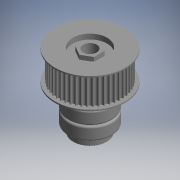
# Autodesk Inventor part: SLZ_63_Riemengetribe#
Saved by Autodesk Inventor 2017.3 (Build 213256000, 256)
## iProperties
Part Number: SLZ_63_Riemengetribe#
Material: Generic
Catalog Web Link: www.cadenas.de
Description: Riemengetr SLZ63-Control-Tec
Vendor: ROSEKRIEGER
Document SubType Name: Modeling
Designer: partserver
Manufacturer: ROSEKRIEGER
Mass: 220.102 g
Surface Area: 442.703 cm^2
Volume: 220.102 cm^3
Density: 1 g/cm^3
Appearance: PSOLRGB-175-175-175
Category: PARTsolutions
Company: ROSEKRIEGER
Title: SLZ_63_Riemengetribe#
Author: Cadenas PARTsolutions
Comments: Control-Tec
PSOL_IDENT_0: {$CADENAS_DATA\23d-libs\rose_krieger\linearkomponenten\pool_lineartechnik\_hubsaeule_zyliinder\elekt
PSOL_IDENT_1: rozylinder\elekzyl_slz63\parts\slz63_plfl_riemengetribe.prj},192 {VTYP=3D},{NB=SLZ_63_Riemengetribe#
PSOL_IDENT_2: },{LINA=SLZ_63_Riemengetribe#},{NN=Riemengetr SLZ63},{DATE=02.12.2020 11:16:20},{GEOMDATE=22.06.2016
PSOL_IDENT_3: 13:04:22},{VERSION=},{LINEID=10},{WBVAR=},{WBNUMERIC=}  {NB=SLZ_63_Riemengetribe#},{LINA=SLZ_63_Rie
PSOL_IDENT_4: mengetribe#},{KT=DUMMY},{IDNR=},{CODE=TQ3},{ARTIKEL=Elektrozylinder },{TYPE=SLZ 63 KG P PL},{BEST=SL
PSOL_IDENT_5: Z_63_Riemengetribe},{VARIANTE=PL},{SPINDEL=KG 25x10},{SPINDELCODE=3.000},{SCHUTZARTVIS=IP54},{SCHUTZ
PSOL_IDENT_6: ART=1},{HUB1=0,[0:100]},{HINWEINBAUX=Hub + 288,5 mm},{DUMMYDURCH=10.000},{DUMMYLAENG=20.000},{HILFEH
PSOL_IDENT_7: UB=105},{LAENDOPPROFIL=184.500},{RF=1.000},{GRUNDKOE=288.500},{A=100},{B=80},{C=100},{D=125},{E=238}
PSOL_IDENT_8: ,{F=40},{G=M16x1.5},{H=104},{K=125},{L=105},{M=48},{N=56.5},{O=86},{P=18.5},{PPATH=sbl_lz70p_plfl.pr
PSOL_IDENT_9: j}
NB: SLZ_63_Riemengetribe#
NN: Riemengetr SLZ63
NT: Control-Tec
NBSYN: $BEST.#
LINA: SLZ_63_Riemengetribe#
CATALOG: RK Rose+Krieger
BEST: SLZ_63_Riemengetribe
VARIANTE: PL
SPINDEL: KG 25x10
SPINDELCODE: 3
SCHUTZARTVIS: IP54
SCHUTZART: 1
HUB1: 0,[0:100]
HINWEINBAUX: Hub + 288,5 mm
HILFEHUB: 105
LAENDOPPROFIL: 184.5
RF: 1
GRUNDKOE: 288.5
A: 100
B: 80
C: 100
D: 125
E: 238
F: 40
G: M16x1.5
H: 104
K: 125
L: 105
M: 48
N: 56.5
O: 86
P: 18.5
SUPPLIER: ROSEKRIEGER
ARTICLENO: SLZ_63_Riemengetribe#
BOMINFO: SLZ_63_Riemengetribe#
CREATOR: CADENAS GmbH
Autodesk Inventor part; units mm, degrees
sketch "Sketch_3" plane through (0, 0, 0) normal (1, 0, 0) x (0, 0, -1)
  line L0 (0, 0) -> (-87, 0)
  line L1 (-87, 19.5) -> (-87, 10)
  line L2 (-87, 10) -> (-36, 10)
  line L3 (-36, 10) -> (-36, 8)
  line L4 (-36, 8) -> (-1, 8)
  line L5 (-1, 8) -> (-1, 12.975)
  line L6 (-1, 12.975) -> (-6, 12.975)
  line L7 (-6, 12.975) -> (-6, 20.25)
  line L8 (-6, 20.25) -> (0, 20.25)
  line L9 (0, 20.25) -> (0, 41.5)
  line L10 (0, 41.5) -> (-1.5, 41.5)
  line L11 (-1.5, 41.5) -> (-1.5, 24)
  line L12 (-1.5, 24) -> (-34.5, 24)
  line L13 (-34.5, 24) -> (-34.5, 41.5)
  line L14 (-34.5, 41.5) -> (-36, 41.5)
  line L15 (-36, 41.5) -> (-36, 20)
  line L16 (-36, 20) -> (-38, 20)
  line L17 (-38, 20) -> (-38, 26)
  line L18 (-38, 26) -> (-39, 27)
  line L19 (-39, 27) -> (-44.5, 27)
  line L20 (-44.5, 27) -> (-45.5, 26)
  line L21 (-45.5, 26) -> (-45.5, 25.5)
  line L22 (-45.5, 25.5) -> (-46.5, 25.5)
  line L23 (-46.5, 25.5) -> (-47, 25)
  line L24 (-47, 25) -> (-47, 24)
  arc A0 (-47, 24) -> (-49, 26) centre (-49, 24) ccw
  line L25 (-49, 26) -> (-60, 26)
  arc A1 (-60, 26) -> (-62, 24) centre (-60, 24) ccw
  line L26 (-62, 24) -> (-62, 20)
  line L27 (-62, 20) -> (-63, 20)
  line L28 (-63, 20) -> (-63, 24)
  arc A2 (-63, 24) -> (-65, 26) centre (-65, 24) ccw
  line L29 (-65, 26) -> (-76, 26)
  arc A3 (-76, 26) -> (-78, 24) centre (-76, 24) ccw
  line L30 (-78, 24) -> (-78, 15)
  line L31 (-78, 15) -> (-79, 15)
  line L32 (-79, 15) -> (-79, 19.5)
  line L33 (-79, 19.5) -> (-79.5, 20)
  line L34 (-79.5, 20) -> (-86.5, 20)
  line L35 (-86.5, 20) -> (-87, 19.5)
  constraints: 72 end point, 8 point on circle, 4 centre point
revolve "Revolution1" add sketch "Sketch_3" angle 360 about axis through (0, 0, 0) along (0, 0, -1)
sketch "Sketch_1" plane through (0, 0, 1.5) normal (0, 0, 1) x (1, 0, 0)
  arc A0 (-37.2613, -1.9994) -> (-37.5535, -2.3178) centre (-37.2541, -2.2993) ccw
  arc A1 (-37.5535, -2.3178) -> (-37.5348, -2.6037) centre (0, 0) ccw
  arc A2 (-37.5348, -2.6037) -> (-37.2035, -2.8812) centre (-37.2355, -2.583) ccw
  arc A3 (-36.6815, -6.8459) -> (-37.2035, -2.8812) centre (-36.9898, -4.8698) ccw
  arc A4 (-36.6815, -6.8459) -> (-36.9297, -7.1997) centre (-36.6353, -7.1423) ccw
  arc A5 (-36.9297, -7.1997) -> (-36.8738, -7.4807) centre (0, 0) ccw
  arc A6 (-36.8738, -7.4807) -> (-36.5091, -7.7126) centre (-36.5798, -7.4211) ccw
  arc A7 (-35.4741, -11.5752) -> (-36.5091, -7.7126) centre (-36.0377, -9.6563) ccw
  arc A8 (-35.4741, -11.5752) -> (-35.674, -11.9584) centre (-35.3896, -11.8631) ccw
  arc A9 (-35.674, -11.9584) -> (-35.5819, -12.2297) centre (0, 0) ccw
  arc A10 (-35.5819, -12.2297) -> (-35.1901, -12.412) centre (-35.2982, -12.1322) ccw
  arc A11 (-33.6598, -16.1065) -> (-35.1901, -12.412) centre (-34.469, -14.2775) ccw
  arc A12 (-33.6598, -16.1065) -> (-33.808, -16.5125) centre (-33.5384, -16.3808) ccw
  arc A13 (-33.808, -16.5125) -> (-33.6812, -16.7695) centre (0, 0) ccw
  arc A14 (-33.6812, -16.7695) -> (-33.2689, -16.8991) centre (-33.4127, -16.6358) ccw
  arc A15 (-31.2695, -20.3622) -> (-33.2689, -16.8991) centre (-32.3105, -18.6545) ccw
  arc A16 (-31.2695, -20.3622) -> (-31.3634, -20.7841) centre (-31.1133, -20.6183) ccw
  arc A17 (-31.3634, -20.7841) -> (-31.2042, -21.0223) centre (0, 0) ccw
  arc A18 (-31.2042, -21.0223) -> (-30.7785, -21.097) centre (-30.9554, -20.8547) ccw
  arc A19 (-28.3442, -24.2695) -> (-30.7785, -21.097) centre (-29.5992, -22.7123) ccw
  arc A20 (-28.3442, -24.2695) -> (-28.3822, -24.7) centre (-28.1559, -24.5031) ccw
  arc A21 (-28.3822, -24.7) -> (-28.1933, -24.9154) centre (0, 0) ccw
  arc A22 (-28.1933, -24.9154) -> (-27.7615, -24.9339) centre (-27.9685, -24.7168) ccw
  arc A23 (-24.9339, -27.7615) -> (-27.7615, -24.9339) centre (-26.3814, -26.3814) ccw
  arc A24 (-24.9339, -27.7615) -> (-24.9154, -28.1933) centre (-24.7168, -27.9685) ccw
  arc A25 (-24.9154, -28.1933) -> (-24.7, -28.3822) centre (0, 0) ccw
  arc A26 (-24.7, -28.3822) -> (-24.2695, -28.3442) centre (-24.5031, -28.1559) ccw
  arc A27 (-21.097, -30.7785) -> (-24.2695, -28.3442) centre (-22.7123, -29.5992) ccw
  arc A28 (-21.097, -30.7785) -> (-21.0223, -31.2042) centre (-20.8547, -30.9554) ccw
  arc A29 (-21.0223, -31.2042) -> (-20.7841, -31.3634) centre (0, 0) ccw
  arc A30 (-20.7841, -31.3634) -> (-20.3622, -31.2695) centre (-20.6183, -31.1133) ccw
  arc A31 (-16.8991, -33.2689) -> (-20.3622, -31.2695) centre (-18.6545, -32.3105) ccw
  arc A32 (-16.8991, -33.2689) -> (-16.7695, -33.6812) centre (-16.6358, -33.4127) ccw
  arc A33 (-16.7695, -33.6812) -> (-16.5125, -33.808) centre (0, 0) ccw
  arc A34 (-16.5125, -33.808) -> (-16.1065, -33.6598) centre (-16.3808, -33.5384) ccw
  arc A35 (-12.412, -35.1901) -> (-16.1065, -33.6598) centre (-14.2775, -34.469) ccw
  arc A36 (-12.412, -35.1901) -> (-12.2297, -35.5819) centre (-12.1322, -35.2982) ccw
  arc A37 (-12.2297, -35.5819) -> (-11.9584, -35.674) centre (0, 0) ccw
  arc A38 (-11.9584, -35.674) -> (-11.5752, -35.4741) centre (-11.8631, -35.3896) ccw
  arc A39 (-7.7126, -36.5091) -> (-11.5752, -35.4741) centre (-9.6563, -36.0377) ccw
  arc A40 (-7.7126, -36.5091) -> (-7.4807, -36.8738) centre (-7.4211, -36.5798) ccw
  arc A41 (-7.4807, -36.8738) -> (-7.1997, -36.9297) centre (0, 0) ccw
  arc A42 (-7.1997, -36.9297) -> (-6.8459, -36.6815) centre (-7.1423, -36.6353) ccw
  arc A43 (-2.8812, -37.2035) -> (-6.8459, -36.6815) centre (-4.8698, -36.9898) ccw
  arc A44 (-2.8812, -37.2035) -> (-2.6037, -37.5348) centre (-2.583, -37.2355) ccw
  arc A45 (-2.6037, -37.5348) -> (-2.3178, -37.5535) centre (0, 0) ccw
  arc A46 (-2.3178, -37.5535) -> (-1.9994, -37.2613) centre (-2.2993, -37.2541) ccw
  arc A47 (1.9994, -37.2613) -> (-1.9994, -37.2613) centre (0, -37.309) ccw
  arc A48 (1.9994, -37.2613) -> (2.3178, -37.5535) centre (2.2993, -37.2541) ccw
  arc A49 (2.3178, -37.5535) -> (2.6037, -37.5348) centre (0, 0) ccw
  arc A50 (2.6037, -37.5348) -> (2.8812, -37.2035) centre (2.583, -37.2355) ccw
  arc A51 (6.8459, -36.6815) -> (2.8812, -37.2035) centre (4.8698, -36.9898) ccw
  arc A52 (6.8459, -36.6815) -> (7.1997, -36.9297) centre (7.1423, -36.6353) ccw
  arc A53 (7.1997, -36.9297) -> (7.4807, -36.8738) centre (0, 0) ccw
  arc A54 (7.4807, -36.8738) -> (7.7126, -36.5091) centre (7.4211, -36.5798) ccw
  arc A55 (11.5752, -35.4741) -> (7.7126, -36.5091) centre (9.6563, -36.0377) ccw
  arc A56 (11.5752, -35.4741) -> (11.9584, -35.674) centre (11.8631, -35.3896) ccw
  arc A57 (11.9584, -35.674) -> (12.2297, -35.5819) centre (0, 0) ccw
  arc A58 (12.2297, -35.5819) -> (12.412, -35.1901) centre (12.1322, -35.2982) ccw
  arc A59 (16.1065, -33.6598) -> (12.412, -35.1901) centre (14.2775, -34.469) ccw
  arc A60 (16.1065, -33.6598) -> (16.5125, -33.808) centre (16.3808, -33.5384) ccw
  arc A61 (16.5125, -33.808) -> (16.7695, -33.6812) centre (0, 0) ccw
  arc A62 (16.7695, -33.6812) -> (16.8991, -33.2689) centre (16.6358, -33.4127) ccw
  arc A63 (20.3622, -31.2695) -> (16.8991, -33.2689) centre (18.6545, -32.3105) ccw
  arc A64 (20.3622, -31.2695) -> (20.7841, -31.3634) centre (20.6183, -31.1133) ccw
  arc A65 (20.7841, -31.3634) -> (21.0223, -31.2042) centre (0, 0) ccw
  arc A66 (21.0223, -31.2042) -> (21.097, -30.7785) centre (20.8547, -30.9554) ccw
  arc A67 (24.2695, -28.3442) -> (21.097, -30.7785) centre (22.7123, -29.5992) ccw
  arc A68 (24.2695, -28.3442) -> (24.7, -28.3822) centre (24.5031, -28.1559) ccw
  arc A69 (24.7, -28.3822) -> (24.9154, -28.1933) centre (0, 0) ccw
  arc A70 (24.9154, -28.1933) -> (24.9339, -27.7615) centre (24.7168, -27.9685) ccw
  arc A71 (27.7615, -24.9339) -> (24.9339, -27.7615) centre (26.3814, -26.3814) ccw
  arc A72 (27.7615, -24.9339) -> (28.1933, -24.9154) centre (27.9685, -24.7168) ccw
  arc A73 (28.1933, -24.9154) -> (28.3822, -24.7) centre (0, 0) ccw
  arc A74 (28.3822, -24.7) -> (28.3442, -24.2695) centre (28.1559, -24.5031) ccw
  arc A75 (30.7785, -21.097) -> (28.3442, -24.2695) centre (29.5992, -22.7123) ccw
  arc A76 (30.7785, -21.097) -> (31.2042, -21.0223) centre (30.9554, -20.8547) ccw
  arc A77 (31.2042, -21.0223) -> (31.3634, -20.7841) centre (0, 0) ccw
  arc A78 (31.3634, -20.7841) -> (31.2695, -20.3622) centre (31.1133, -20.6183) ccw
  arc A79 (33.2689, -16.8991) -> (31.2695, -20.3622) centre (32.3105, -18.6545) ccw
  arc A80 (33.2689, -16.8991) -> (33.6812, -16.7695) centre (33.4127, -16.6358) ccw
  arc A81 (33.6812, -16.7695) -> (33.808, -16.5125) centre (0, 0) ccw
  arc A82 (33.808, -16.5125) -> (33.6598, -16.1065) centre (33.5384, -16.3808) ccw
  arc A83 (35.1901, -12.412) -> (33.6598, -16.1065) centre (34.469, -14.2775) ccw
  arc A84 (35.1901, -12.412) -> (35.5819, -12.2297) centre (35.2982, -12.1322) ccw
  arc A85 (35.5819, -12.2297) -> (35.674, -11.9584) centre (0, 0) ccw
  arc A86 (35.674, -11.9584) -> (35.4741, -11.5752) centre (35.3896, -11.8631) ccw
  arc A87 (36.5091, -7.7126) -> (35.4741, -11.5752) centre (36.0377, -9.6563) ccw
  arc A88 (36.5091, -7.7126) -> (36.8738, -7.4807) centre (36.5798, -7.4211) ccw
  arc A89 (36.8738, -7.4807) -> (36.9297, -7.1997) centre (0, 0) ccw
  arc A90 (36.9297, -7.1997) -> (36.6815, -6.8459) centre (36.6353, -7.1423) ccw
  arc A91 (37.2035, -2.8812) -> (36.6815, -6.8459) centre (36.9898, -4.8698) ccw
  arc A92 (37.2035, -2.8812) -> (37.5348, -2.6037) centre (37.2355, -2.583) ccw
  arc A93 (37.5348, -2.6037) -> (37.5535, -2.3178) centre (0, 0) ccw
  arc A94 (37.5535, -2.3178) -> (37.2613, -1.9994) centre (37.2541, -2.2993) ccw
  arc A95 (37.2613, 1.9994) -> (37.2613, -1.9994) centre (37.309, 0) ccw
  arc A96 (37.2613, 1.9994) -> (37.5535, 2.3178) centre (37.2541, 2.2993) ccw
  arc A97 (37.5535, 2.3178) -> (37.5348, 2.6037) centre (0, 0) ccw
  arc A98 (37.5348, 2.6037) -> (37.2035, 2.8812) centre (37.2355, 2.583) ccw
  arc A99 (36.6815, 6.8459) -> (37.2035, 2.8812) centre (36.9898, 4.8698) ccw
  arc A100 (36.6815, 6.8459) -> (36.9297, 7.1997) centre (36.6353, 7.1423) ccw
  arc A101 (36.9297, 7.1997) -> (36.8738, 7.4807) centre (0, 0) ccw
  arc A102 (36.8738, 7.4807) -> (36.5091, 7.7126) centre (36.5798, 7.4211) ccw
  arc A103 (35.4741, 11.5752) -> (36.5091, 7.7126) centre (36.0377, 9.6563) ccw
  arc A104 (35.4741, 11.5752) -> (35.674, 11.9584) centre (35.3896, 11.8631) ccw
  arc A105 (35.674, 11.9584) -> (35.5819, 12.2297) centre (0, 0) ccw
  arc A106 (35.5819, 12.2297) -> (35.1901, 12.412) centre (35.2982, 12.1322) ccw
  arc A107 (33.6598, 16.1065) -> (35.1901, 12.412) centre (34.469, 14.2775) ccw
  arc A108 (33.6598, 16.1065) -> (33.808, 16.5125) centre (33.5384, 16.3808) ccw
  arc A109 (33.808, 16.5125) -> (33.6812, 16.7695) centre (0, 0) ccw
  arc A110 (33.6812, 16.7695) -> (33.2689, 16.8991) centre (33.4127, 16.6358) ccw
  arc A111 (31.2695, 20.3622) -> (33.2689, 16.8991) centre (32.3105, 18.6545) ccw
  arc A112 (31.2695, 20.3622) -> (31.3634, 20.7841) centre (31.1133, 20.6183) ccw
  arc A113 (31.3634, 20.7841) -> (31.2042, 21.0223) centre (0, 0) ccw
  arc A114 (31.2042, 21.0223) -> (30.7785, 21.097) centre (30.9554, 20.8547) ccw
  arc A115 (28.3442, 24.2695) -> (30.7785, 21.097) centre (29.5992, 22.7123) ccw
  arc A116 (28.3442, 24.2695) -> (28.3822, 24.7) centre (28.1559, 24.5031) ccw
  arc A117 (28.3822, 24.7) -> (28.1933, 24.9154) centre (0, 0) ccw
  arc A118 (28.1933, 24.9154) -> (27.7615, 24.9339) centre (27.9685, 24.7168) ccw
  arc A119 (24.9339, 27.7615) -> (27.7615, 24.9339) centre (26.3814, 26.3814) ccw
  arc A120 (24.9339, 27.7615) -> (24.9154, 28.1933) centre (24.7168, 27.9685) ccw
  arc A121 (24.9154, 28.1933) -> (24.7, 28.3822) centre (0, 0) ccw
  arc A122 (24.7, 28.3822) -> (24.2695, 28.3442) centre (24.5031, 28.1559) ccw
  arc A123 (21.097, 30.7785) -> (24.2695, 28.3442) centre (22.7123, 29.5992) ccw
  arc A124 (21.097, 30.7785) -> (21.0223, 31.2042) centre (20.8547, 30.9554) ccw
  arc A125 (21.0223, 31.2042) -> (20.7841, 31.3634) centre (0, 0) ccw
  arc A126 (20.7841, 31.3634) -> (20.3622, 31.2695) centre (20.6183, 31.1133) ccw
  arc A127 (16.8991, 33.2689) -> (20.3622, 31.2695) centre (18.6545, 32.3105) ccw
  arc A128 (16.8991, 33.2689) -> (16.7695, 33.6812) centre (16.6358, 33.4127) ccw
  arc A129 (16.7695, 33.6812) -> (16.5125, 33.808) centre (0, 0) ccw
  arc A130 (16.5125, 33.808) -> (16.1065, 33.6598) centre (16.3808, 33.5384) ccw
  arc A131 (12.412, 35.1901) -> (16.1065, 33.6598) centre (14.2775, 34.469) ccw
  arc A132 (12.412, 35.1901) -> (12.2297, 35.5819) centre (12.1322, 35.2982) ccw
  arc A133 (12.2297, 35.5819) -> (11.9584, 35.674) centre (0, 0) ccw
  arc A134 (11.9584, 35.674) -> (11.5752, 35.4741) centre (11.8631, 35.3896) ccw
  arc A135 (7.7126, 36.5091) -> (11.5752, 35.4741) centre (9.6563, 36.0377) ccw
  arc A136 (7.7126, 36.5091) -> (7.4807, 36.8738) centre (7.4211, 36.5798) ccw
  arc A137 (7.4807, 36.8738) -> (7.1997, 36.9297) centre (0, 0) ccw
  arc A138 (7.1997, 36.9297) -> (6.8459, 36.6815) centre (7.1423, 36.6353) ccw
  arc A139 (2.8812, 37.2035) -> (6.8459, 36.6815) centre (4.8698, 36.9898) ccw
  arc A140 (2.8812, 37.2035) -> (2.6037, 37.5348) centre (2.583, 37.2355) ccw
  arc A141 (2.6037, 37.5348) -> (2.3178, 37.5535) centre (0, 0) ccw
  arc A142 (2.3178, 37.5535) -> (1.9994, 37.2613) centre (2.2993, 37.2541) ccw
  arc A143 (-1.9994, 37.2613) -> (1.9994, 37.2613) centre (0, 37.309) ccw
  arc A144 (-1.9994, 37.2613) -> (-2.3178, 37.5535) centre (-2.2993, 37.2541) ccw
  arc A145 (-2.3178, 37.5535) -> (-2.6037, 37.5348) centre (0, 0) ccw
  arc A146 (-2.6037, 37.5348) -> (-2.8812, 37.2035) centre (-2.583, 37.2355) ccw
  arc A147 (-6.8459, 36.6815) -> (-2.8812, 37.2035) centre (-4.8698, 36.9898) ccw
  arc A148 (-6.8459, 36.6815) -> (-7.1997, 36.9297) centre (-7.1423, 36.6353) ccw
  arc A149 (-7.1997, 36.9297) -> (-7.4807, 36.8738) centre (0, 0) ccw
  arc A150 (-7.4807, 36.8738) -> (-7.7126, 36.5091) centre (-7.4211, 36.5798) ccw
  arc A151 (-11.5752, 35.4741) -> (-7.7126, 36.5091) centre (-9.6563, 36.0377) ccw
  arc A152 (-11.5752, 35.4741) -> (-11.9584, 35.674) centre (-11.8631, 35.3896) ccw
  arc A153 (-11.9584, 35.674) -> (-12.2297, 35.5819) centre (0, 0) ccw
  arc A154 (-12.2297, 35.5819) -> (-12.412, 35.1901) centre (-12.1322, 35.2982) ccw
  arc A155 (-16.1065, 33.6598) -> (-12.412, 35.1901) centre (-14.2775, 34.469) ccw
  arc A156 (-16.1065, 33.6598) -> (-16.5125, 33.808) centre (-16.3808, 33.5384) ccw
  arc A157 (-16.5125, 33.808) -> (-16.7695, 33.6812) centre (0, 0) ccw
  arc A158 (-16.7695, 33.6812) -> (-16.8991, 33.2689) centre (-16.6358, 33.4127) ccw
  arc A159 (-20.3622, 31.2695) -> (-16.8991, 33.2689) centre (-18.6545, 32.3105) ccw
  arc A160 (-20.3622, 31.2695) -> (-20.7841, 31.3634) centre (-20.6183, 31.1133) ccw
  arc A161 (-20.7841, 31.3634) -> (-21.0223, 31.2042) centre (0, 0) ccw
  arc A162 (-21.0223, 31.2042) -> (-21.097, 30.7785) centre (-20.8547, 30.9554) ccw
  arc A163 (-24.2695, 28.3442) -> (-21.097, 30.7785) centre (-22.7123, 29.5992) ccw
  arc A164 (-24.2695, 28.3442) -> (-24.7, 28.3822) centre (-24.5031, 28.1559) ccw
  arc A165 (-24.7, 28.3822) -> (-24.9154, 28.1933) centre (0, 0) ccw
  arc A166 (-24.9154, 28.1933) -> (-24.9339, 27.7615) centre (-24.7168, 27.9685) ccw
  arc A167 (-27.7615, 24.9339) -> (-24.9339, 27.7615) centre (-26.3814, 26.3814) ccw
  arc A168 (-27.7615, 24.9339) -> (-28.1933, 24.9154) centre (-27.9685, 24.7168) ccw
  arc A169 (-28.1933, 24.9154) -> (-28.3822, 24.7) centre (0, 0) ccw
  arc A170 (-28.3822, 24.7) -> (-28.3442, 24.2695) centre (-28.1559, 24.5031) ccw
  arc A171 (-30.7785, 21.097) -> (-28.3442, 24.2695) centre (-29.5992, 22.7123) ccw
  arc A172 (-30.7785, 21.097) -> (-31.2042, 21.0223) centre (-30.9554, 20.8547) ccw
  arc A173 (-31.2042, 21.0223) -> (-31.3634, 20.7841) centre (0, 0) ccw
  arc A174 (-31.3634, 20.7841) -> (-31.2695, 20.3622) centre (-31.1133, 20.6183) ccw
  arc A175 (-33.2689, 16.8991) -> (-31.2695, 20.3622) centre (-32.3105, 18.6545) ccw
  arc A176 (-33.2689, 16.8991) -> (-33.6812, 16.7695) centre (-33.4127, 16.6358) ccw
  arc A177 (-33.6812, 16.7695) -> (-33.808, 16.5125) centre (0, 0) ccw
  arc A178 (-33.808, 16.5125) -> (-33.6598, 16.1065) centre (-33.5384, 16.3808) ccw
  arc A179 (-35.1901, 12.412) -> (-33.6598, 16.1065) centre (-34.469, 14.2775) ccw
  arc A180 (-35.1901, 12.412) -> (-35.5819, 12.2297) centre (-35.2982, 12.1322) ccw
  arc A181 (-35.5819, 12.2297) -> (-35.674, 11.9584) centre (0, 0) ccw
  arc A182 (-35.674, 11.9584) -> (-35.4741, 11.5752) centre (-35.3896, 11.8631) ccw
  arc A183 (-36.5091, 7.7126) -> (-35.4741, 11.5752) centre (-36.0377, 9.6563) ccw
  arc A184 (-36.5091, 7.7126) -> (-36.8738, 7.4807) centre (-36.5798, 7.4211) ccw
  arc A185 (-36.8738, 7.4807) -> (-36.9297, 7.1997) centre (0, 0) ccw
  arc A186 (-36.9297, 7.1997) -> (-36.6815, 6.8459) centre (-36.6353, 7.1423) ccw
  arc A187 (-37.2035, 2.8812) -> (-36.6815, 6.8459) centre (-36.9898, 4.8698) ccw
  arc A188 (-37.2035, 2.8812) -> (-37.5348, 2.6037) centre (-37.2355, 2.583) ccw
  arc A189 (-37.5348, 2.6037) -> (-37.5535, 2.3178) centre (0, 0) ccw
  arc A190 (-37.5535, 2.3178) -> (-37.2613, 1.9994) centre (-37.2541, 2.2993) ccw
  arc A191 (-37.2613, -1.9994) -> (-37.2613, 1.9994) centre (-37.309, 0) ccw
  circle A192 centre (0, 0) radius 23
  constraints: 384 point on circle, 193 centre point
extrude "Extrusion1" add sketch "Sketch_1" along normal blind 33
sketch "Sketch_4" plane through (0, 0, 0) normal (0, 0, 1) x (1, 0, 0)
  circle A0 centre (0, 0) radius 20
  line L0 (-11, -6.3509) -> (0, -12.7017)
  line L1 (0, -12.7017) -> (11, -6.3509)
  line L2 (11, -6.3509) -> (11, 6.3509)
  line L3 (11, 6.3509) -> (0, 12.7017)
  line L4 (0, 12.7017) -> (-11, 6.3509)
  line L5 (-11, 6.3509) -> (-11, -6.3509)
  constraints: 12 end point, 1 centre point
extrude "Extrusion2" cut sketch "Sketch_4" along normal blind 6
ref_plane "RIEMEN_XY" through (0, 0, 18) normal (0, 0, 1) x (1, 0, 0)
ref_plane "RIEMEN_YZ" through (0, 0, 18) normal (1, 0, 0) x (0, 1, 0)
ref_plane "RIEMEN_ZX" through (0, 0, 18) normal (0, 1, 0) x (0, 0, 1)
ref_plane "RIEMENGETRIBE_XY" through (0, 0, 0) normal (0, 0, -1) x (1, 0, 0)
ref_plane "RIEMENGETRIBE_YZ" through (0, 0, 0) normal (1, 0, 0) x (0, -1, 0)
ref_plane "RIEMENGETRIBE_ZX" through (0, 0, 0) normal (0, -1, 0) x (0, 0, -1)
body "Solid1"
